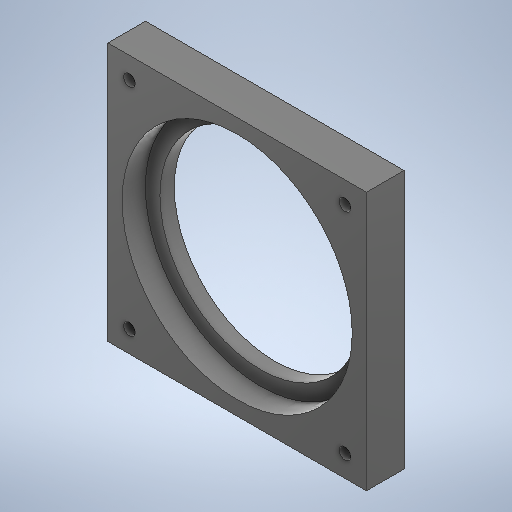
# Autodesk Inventor part: bearing_bracket1
Saved by Autodesk Inventor 2026.2 (Build 302298010, 298A)
## iProperties
Created: 2026-04-11
Part Number: bearing_bracket1
Material: ABS Plastic
Document SubType Name: Modeling
Designer: chris
Density: 1.06 g/cm^3
Appearance: Smooth - White
Author: chris
Autodesk Inventor part; units mm, degrees
ref_plane "YZ Plane" through (0, 0, 0) normal (1, 0, 0) x (0, 1, 0)
ref_plane "XZ Plane" through (0, 0, 0) normal (0, 1, 0) x (-1, 0, 0)
ref_plane "XY Plane" through (0, 0, 0) normal (0, 0, 1) x (1, 0, 0)
sketch "Sketch4" plane through (0, 0, 0) normal (0, 0, 1) x (1, 0, 0)
  line L0 (-45, -45) -> (45, -45)
  line L1 (45, -45) -> (45, 45)
  line L2 (45, 45) -> (-45, 45)
  line L3 (-45, 45) -> (-45, -45)
  line L4 (-45, -45) -> (45, 45) construction
  line L5 (45, -45) -> (-45, 45) construction
  point P0 (0, 0)
  dimension "d10" = 90
  dimension "d11" = 90
  constraints: 12 end point, 2 midpoint, 2 parallel, 1 horizontal, 1 perpendicular
  measures "d10" distance of L1.end L2.end
  measures "d11" distance of L0.end L1.end
extrude "Extrusion4" add sketch "Sketch4" along normal blind 5
sketch "Sketch5" plane through (0, 0, 5) normal (0, 0, 1) x (1, 0, 0)
  line L0 (-45, -45) -> (45, -45)
  line L1 (45, -45) -> (45, 45)
  line L2 (45, 45) -> (-45, 45)
  line L3 (-45, 45) -> (-45, -45)
  line L4 (-45, -45) -> (45, 45) construction
  line L5 (45, -45) -> (-45, 45) construction
  line L6 (45, 45) -> (-45, 45) projected
  line L7 (45, -45) -> (45, 45) projected
  circle A0 centre (0, 0) radius 40.05
  dimension "d14" = 80.1
  constraints: 12 end point, 2 collinear, 2 midpoint, 2 parallel, 1 centre point, 1 coincident, 1 horizontal, 1 perpendicular
  measures "d14" diameter of A0
extrude "Extrusion5" add sketch "Sketch5" along normal blind 8.1
sketch "Sketch6" plane through (0, 0, 5) normal (0, 0, 1) x (1, 0, 0)
  circle A0 centre (0, 0) radius 35
  dimension "d17" = 70
  constraints: 1 centre point, 1 coincident
  measures "d17" diameter of A0
extrude "Extrusion6" cut sketch "Sketch6" against normal through all
sketch "Sketch7" plane through (0, 0, 0) normal (0, 0, -1) x (-1, 0, 0)
  circle A0 centre (-37.5, -37.5) radius 2.05
  circle A1 centre (-37.5, 37.5) radius 2.05
  circle A2 centre (37.5, 37.5) radius 2.05
  circle A3 centre (37.5, -37.5) radius 2.05
  line L0 (-45, -45) -> (-45, 45) projected
  line L1 (45, -45) -> (-45, -45) projected
  line L2 (-45, 45) -> (45, 45) projected
  line L3 (45, 45) -> (45, -45) projected
  point P0 (0, 0)
  dimension "d20" = 4.1
  dimension "d21" = 4.1
  dimension "d22" = 4.1
  dimension "d23" = 4.1
  dimension "d24" = 7.5
  dimension "d25" = 7.5
  dimension "d26" = 7.5
  dimension "d27" = 7.5
  dimension "d28" = 7.5
  dimension "d29" = 7.5
  dimension "d30" = 7.5
  dimension "d31" = 7.5
  constraints: 4 centre point
  measures "d20" diameter of A0
  measures "d21" diameter of A1
  measures "d22" diameter of A2
  measures "d23" diameter of A3
  measures "d24" distance from line of L0 A0.centre
  measures "d25" distance from line of L1 A0.centre
  measures "d26" distance from line of L0 A1.centre
  measures "d27" distance from line of L2 A1.centre
  measures "d28" distance from line of L2 A2.centre
  measures "d29" distance from line of L3 A2.centre
  measures "d30" distance from line of L3 A3.centre
  measures "d31" distance from line of L1 A3.centre
extrude "Extrusion7" cut sketch "Sketch7" against normal through all contours A0 | A1 | A2 | A3
sketch "Sketch8" plane through (0, 0, 0) normal (0, 0, -1) x (-1, 0, 0)
  circle A0 centre (-37.5, -37.5) radius 2.05 projected
  circle A1 centre (-37.5, 37.5) radius 2.05 projected
  circle A2 centre (37.5, 37.5) radius 2.05 projected
  circle A3 centre (37.5, -37.5) radius 2.05 projected
  circle A4 centre (-37.5, -37.5) radius 5
  circle A5 centre (-37.5, 37.5) radius 5
  circle A6 centre (37.5, 37.5) radius 5
  circle A7 centre (37.5, -37.5) radius 5
  point P0 (0, 0)
  dimension "d34" = 10
  dimension "d35" = 10
  dimension "d36" = 10
  dimension "d37" = 10
  constraints: 4 centre point, 4 coincident
  measures "d34" diameter of A4
  measures "d35" diameter of A5
  measures "d36" diameter of A6
  measures "d37" diameter of A7
extrude "Extrusion8" cut sketch "Sketch8" against normal blind 7 contours A1 | A2 | A4 | A5 | A6 | A7
body "Solid2"
